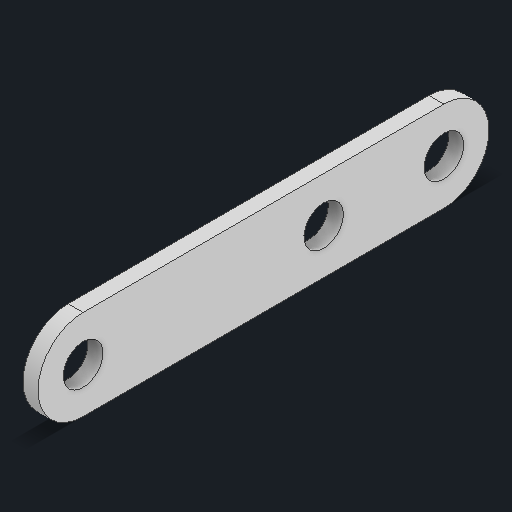
# Autodesk Inventor part: Gearbox Gusset
Saved by Autodesk Inventor 2025.1 (Build 291241000, 241)
## iProperties
Created: 2024-11-06
Part Number: Gearbox Gusset
Material: Generic
Document SubType Name: Modeling
Designer: avere
Density: 1 g/cm^3
Appearance: Default
Author: avere
Autodesk Inventor part; units mm, degrees
ref_plane "YZ Plane" through (0, 0, 0) normal (1, 0, 0) x (0, 1, 0)
ref_plane "XZ Plane" through (0, 0, 0) normal (0, 1, 0) x (-1, 0, 0)
ref_plane "XY Plane" through (0, 0, 0) normal (0, 0, 1) x (1, 0, 0)
sketch "Sketch1" plane through (0, 0, 0) normal (1, 0, 0) x (0, 1, 0)
  circle A0 centre (0, 0) radius 2.1
  circle A1 centre (0, -25.4) radius 2.0828
  circle A2 centre (0, -38.1) radius 2.1
  arc A3 (4.7625, 0) -> (-4.7625, 0) centre (0, 0) ccw
  arc A4 (-4.7625, -38.1) -> (4.7625, -38.1) centre (0, -38.1) ccw
  line L0 (4.7625, 0) -> (4.7625, -38.1)
  line L1 (-4.7625, 0) -> (-4.7625, -38.1)
  dimension "d0" = 4.2
  dimension "d4" = 4.1656
  dimension "d5" = 4.2
  constraints: 5 centre point, 4 end point, 4 point on circle, 3 coincident, 1 parallel, 1 tangent
  measures "d0" diameter of A0
  measures "d4" diameter of A1
  measures "d5" diameter of A2
extrude "Extrusion1" add sketch "Sketch1" along normal blind 1.5875
body "Solid1"
